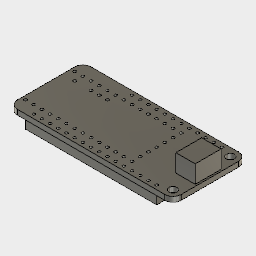
3200 Teensy Feather Adapter (Autodesk Fusion 360 design; units mm, degrees)
Autodesk Fusion 360 part; units mm, degrees
sketch "Adafruit Feather Teensy3 Adapter" plane through (0, 0, 0) normal (0, 0, 1) x (1, 0, 0)
  arc A0 (2.54, 22.86) -> (0, 20.32) centre (2.54, 20.32) ccw
  line L0 (2.54, 0) -> (48.26, 0)
  arc A1 (48.26, 0) -> (50.8, 2.54) centre (48.26, 2.54) ccw
  line L1 (48.26, 22.86) -> (2.54, 22.86)
  arc A2 (0, 2.54) -> (2.54, 0) centre (2.54, 2.54) ccw
  line L2 (0, 20.32) -> (0, 2.54)
  arc A3 (50.8, 20.32) -> (48.26, 22.86) centre (48.26, 20.32) ccw
  line L3 (50.8, 2.54) -> (50.8, 20.32)
  arc A4 (14.4145, 3.81) -> (13.5255, 3.81) centre (13.97, 3.81) ccw
  arc A5 (34.7345, 16.51) -> (33.8455, 16.51) centre (34.29, 16.51) ccw
  arc A6 (32.1945, 3.81) -> (31.3055, 3.81) centre (31.75, 3.81) ccw
  arc A7 (31.3055, 3.81) -> (32.1945, 3.81) centre (31.75, 3.81) ccw
  arc A8 (16.9545, 19.05) -> (16.0655, 19.05) centre (16.51, 19.05) ccw
  arc A9 (37.2491, 1.27) -> (36.4109, 1.27) centre (36.83, 1.27) ccw
  arc A10 (42.3291, 21.59) -> (41.4909, 21.59) centre (41.91, 21.59) ccw
  arc A11 (14.4145, 19.05) -> (13.5255, 19.05) centre (13.97, 19.05) ccw
  arc A12 (26.2255, 19.05) -> (27.1145, 19.05) centre (26.67, 19.05) ccw
  arc A13 (10.9855, 3.81) -> (11.8745, 3.81) centre (11.43, 3.81) ccw
  arc A14 (32.1945, 19.05) -> (31.3055, 19.05) centre (31.75, 19.05) ccw
  arc A15 (3.3655, 16.51) -> (4.2545, 16.51) centre (3.81, 16.51) ccw
  arc A16 (41.4909, 1.27) -> (42.3291, 1.27) centre (41.91, 1.27) ccw
  arc A17 (32.1691, 21.59) -> (31.3309, 21.59) centre (31.75, 21.59) ccw
  arc A18 (33.8709, 21.59) -> (34.7091, 21.59) centre (34.29, 21.59) ccw
  arc A19 (5.9055, 19.05) -> (6.7945, 19.05) centre (6.35, 19.05) ccw
  arc A20 (10.9855, 19.05) -> (11.8745, 19.05) centre (11.43, 19.05) ccw
  arc A21 (36.4109, 21.59) -> (37.2491, 21.59) centre (36.83, 21.59) ccw
  arc A22 (19.4691, 1.27) -> (18.6309, 1.27) centre (19.05, 1.27) ccw
  arc A23 (34.7345, 19.05) -> (33.8455, 19.05) centre (34.29, 19.05) ccw
  arc A24 (39.7891, 21.59) -> (38.9509, 21.59) centre (39.37, 21.59) ccw
  arc A25 (24.5491, 21.59) -> (23.7109, 21.59) centre (24.13, 21.59) ccw
  arc A26 (5.9309, 1.27) -> (6.7691, 1.27) centre (6.35, 1.27) ccw
  arc A27 (39.7891, 1.27) -> (38.9509, 1.27) centre (39.37, 1.27) ccw
  arc A28 (37.2491, 21.59) -> (36.4109, 21.59) centre (36.83, 21.59) ccw
  arc A29 (21.1455, 3.81) -> (22.0345, 3.81) centre (21.59, 3.81) ccw
  arc A30 (29.6545, 3.81) -> (28.7655, 3.81) centre (29.21, 3.81) ccw
  arc A31 (31.3055, 19.05) -> (32.1945, 19.05) centre (31.75, 19.05) ccw
  arc A32 (22.0091, 21.59) -> (21.1709, 21.59) centre (21.59, 21.59) ccw
  arc A33 (18.6309, 21.59) -> (19.4691, 21.59) centre (19.05, 21.59) ccw
  arc A34 (16.9291, 21.59) -> (16.0909, 21.59) centre (16.51, 21.59) ccw
  arc A35 (4.2545, 3.81) -> (3.3655, 3.81) centre (3.81, 3.81) ccw
  arc A36 (19.4691, 21.59) -> (18.6309, 21.59) centre (19.05, 21.59) ccw
  arc A37 (16.0909, 21.59) -> (16.9291, 21.59) centre (16.51, 21.59) ccw
  arc A38 (10.9855, 3.81) -> (11.8745, 3.81) centre (11.43, 3.81) ccw
  arc A39 (32.1691, 1.27) -> (31.3309, 1.27) centre (31.75, 1.27) ccw
  arc A40 (21.1709, 1.27) -> (22.0091, 1.27) centre (21.59, 1.27) ccw
  arc A41 (44.0309, 21.59) -> (44.8691, 21.59) centre (44.45, 21.59) ccw
  arc A42 (18.6055, 3.81) -> (19.4945, 3.81) centre (19.05, 3.81) ccw
  arc A43 (39.7891, 21.59) -> (38.9509, 21.59) centre (39.37, 21.59) ccw
  arc A44 (1.7145, 19.05) -> (0.8255, 19.05) centre (1.27, 19.05) ccw
  arc A45 (31.3055, 19.05) -> (32.1945, 19.05) centre (31.75, 19.05) ccw
  arc A46 (28.7909, 21.59) -> (29.6291, 21.59) centre (29.21, 21.59) ccw
  arc A47 (34.7091, 1.27) -> (33.8709, 1.27) centre (34.29, 1.27) ccw
  arc A48 (34.7091, 1.27) -> (33.8709, 1.27) centre (34.29, 1.27) ccw
  arc A49 (4.2545, 3.81) -> (3.3655, 3.81) centre (3.81, 3.81) ccw
  arc A50 (31.3309, 1.27) -> (32.1691, 1.27) centre (31.75, 1.27) ccw
  arc A51 (28.7909, 1.27) -> (29.6291, 1.27) centre (29.21, 1.27) ccw
  arc A52 (26.2509, 21.59) -> (27.0891, 21.59) centre (26.67, 21.59) ccw
  arc A53 (23.7109, 1.27) -> (24.5491, 1.27) centre (24.13, 1.27) ccw
  arc A54 (33.8455, 8.89) -> (34.7345, 8.89) centre (34.29, 8.89) ccw
  arc A55 (28.7909, 1.27) -> (29.6291, 1.27) centre (29.21, 1.27) ccw
  arc A56 (3.3655, 3.81) -> (4.2545, 3.81) centre (3.81, 3.81) ccw
  arc A57 (29.6291, 21.59) -> (28.7909, 21.59) centre (29.21, 21.59) ccw
  arc A58 (13.5509, 1.27) -> (14.3891, 1.27) centre (13.97, 1.27) ccw
  arc A59 (16.9291, 21.59) -> (16.0909, 21.59) centre (16.51, 21.59) ccw
  arc A60 (27.0891, 1.27) -> (26.2509, 1.27) centre (26.67, 1.27) ccw
  arc A61 (34.7345, 8.89) -> (33.8455, 8.89) centre (34.29, 8.89) ccw
  arc A62 (22.0091, 1.27) -> (21.1709, 1.27) centre (21.59, 1.27) ccw
  arc A63 (9.3345, 3.81) -> (8.4455, 3.81) centre (8.89, 3.81) ccw
  arc A64 (44.8691, 1.27) -> (44.0309, 1.27) centre (44.45, 1.27) ccw
  arc A65 (18.6309, 1.27) -> (19.4691, 1.27) centre (19.05, 1.27) ccw
  arc A66 (33.8709, 1.27) -> (34.7091, 1.27) centre (34.29, 1.27) ccw
  arc A67 (22.0091, 21.59) -> (21.1709, 21.59) centre (21.59, 21.59) ccw
  arc A68 (9.3091, 1.27) -> (8.4709, 1.27) centre (8.89, 1.27) ccw
  arc A69 (16.9291, 1.27) -> (16.0909, 1.27) centre (16.51, 1.27) ccw
  arc A70 (14.3891, 1.27) -> (13.5509, 1.27) centre (13.97, 1.27) ccw
  arc A71 (24.5491, 21.59) -> (23.7109, 21.59) centre (24.13, 21.59) ccw
  arc A72 (23.7109, 1.27) -> (24.5491, 1.27) centre (24.13, 1.27) ccw
  arc A73 (38.9509, 1.27) -> (39.7891, 1.27) centre (39.37, 1.27) ccw
  arc A74 (26.2509, 1.27) -> (27.0891, 1.27) centre (26.67, 1.27) ccw
  arc A75 (16.0909, 1.27) -> (16.9291, 1.27) centre (16.51, 1.27) ccw
  arc A76 (24.5491, 1.27) -> (23.7109, 1.27) centre (24.13, 1.27) ccw
  arc A77 (11.0109, 1.27) -> (11.8491, 1.27) centre (11.43, 1.27) ccw
  arc A78 (44.8691, 21.59) -> (44.0309, 21.59) centre (44.45, 21.59) ccw
  arc A79 (27.0891, 21.59) -> (26.2509, 21.59) centre (26.67, 21.59) ccw
  arc A80 (16.9291, 1.27) -> (16.0909, 1.27) centre (16.51, 1.27) ccw
  arc A81 (21.1709, 1.27) -> (22.0091, 1.27) centre (21.59, 1.27) ccw
  arc A82 (8.4709, 1.27) -> (9.3091, 1.27) centre (8.89, 1.27) ccw
  arc A83 (14.3891, 1.27) -> (13.5509, 1.27) centre (13.97, 1.27) ccw
  arc A84 (29.6291, 21.59) -> (28.7909, 21.59) centre (29.21, 21.59) ccw
  arc A85 (11.8745, 3.81) -> (10.9855, 3.81) centre (11.43, 3.81) ccw
  arc A86 (36.4109, 1.27) -> (37.2491, 1.27) centre (36.83, 1.27) ccw
  arc A87 (33.8455, 8.89) -> (34.7345, 8.89) centre (34.29, 8.89) ccw
  arc A88 (13.5509, 1.27) -> (14.3891, 1.27) centre (13.97, 1.27) ccw
  arc A89 (27.0891, 1.27) -> (26.2509, 1.27) centre (26.67, 1.27) ccw
  arc A90 (23.7109, 21.59) -> (24.5491, 21.59) centre (24.13, 21.59) ccw
  arc A91 (11.0109, 1.27) -> (11.8491, 1.27) centre (11.43, 1.27) ccw
  arc A92 (37.2491, 1.27) -> (36.4109, 1.27) centre (36.83, 1.27) ccw
  arc A93 (29.6291, 1.27) -> (28.7909, 1.27) centre (29.21, 1.27) ccw
  arc A94 (18.6309, 21.59) -> (19.4691, 21.59) centre (19.05, 21.59) ccw
  arc A95 (27.0891, 21.59) -> (26.2509, 21.59) centre (26.67, 21.59) ccw
  arc A96 (5.9309, 1.27) -> (6.7691, 1.27) centre (6.35, 1.27) ccw
  arc A97 (41.4909, 1.27) -> (42.3291, 1.27) centre (41.91, 1.27) ccw
  arc A98 (34.7345, 8.89) -> (33.8455, 8.89) centre (34.29, 8.89) ccw
  arc A99 (29.6291, 1.27) -> (28.7909, 1.27) centre (29.21, 1.27) ccw
  arc A100 (6.7691, 1.27) -> (5.9309, 1.27) centre (6.35, 1.27) ccw
  arc A101 (21.1709, 21.59) -> (22.0091, 21.59) centre (21.59, 21.59) ccw
  arc A102 (6.7691, 1.27) -> (5.9309, 1.27) centre (6.35, 1.27) ccw
  arc A103 (8.4709, 1.27) -> (9.3091, 1.27) centre (8.89, 1.27) ccw
  arc A104 (16.0909, 1.27) -> (16.9291, 1.27) centre (16.51, 1.27) ccw
  arc A105 (9.3091, 1.27) -> (8.4709, 1.27) centre (8.89, 1.27) ccw
  arc A106 (33.8455, 11.43) -> (34.7345, 11.43) centre (34.29, 11.43) ccw
  arc A107 (0.8255, 19.05) -> (1.7145, 19.05) centre (1.27, 19.05) ccw
  arc A108 (16.0655, 19.05) -> (16.9545, 19.05) centre (16.51, 19.05) ccw
  arc A109 (33.8455, 13.97) -> (34.7345, 13.97) centre (34.29, 13.97) ccw
  arc A110 (5.9055, 3.81) -> (6.7945, 3.81) centre (6.35, 3.81) ccw
  arc A111 (16.0655, 3.81) -> (16.9545, 3.81) centre (16.51, 3.81) ccw
  arc A112 (11.8491, 1.27) -> (11.0109, 1.27) centre (11.43, 1.27) ccw
  arc A113 (9.3345, 19.05) -> (8.4455, 19.05) centre (8.89, 19.05) ccw
  arc A114 (44.0309, 1.27) -> (44.8691, 1.27) centre (44.45, 1.27) ccw
  arc A115 (26.2509, 1.27) -> (27.0891, 1.27) centre (26.67, 1.27) ccw
  arc A116 (39.7891, 1.27) -> (38.9509, 1.27) centre (39.37, 1.27) ccw
  arc A117 (22.0345, 19.05) -> (21.1455, 19.05) centre (21.59, 19.05) ccw
  arc A118 (33.8455, 6.35) -> (34.7345, 6.35) centre (34.29, 6.35) ccw
  arc A119 (34.7091, 21.59) -> (33.8709, 21.59) centre (34.29, 21.59) ccw
  arc A120 (32.1691, 1.27) -> (31.3309, 1.27) centre (31.75, 1.27) ccw
  arc A121 (13.5255, 16.51) -> (14.4145, 16.51) centre (13.97, 16.51) ccw
  arc A122 (31.3309, 1.27) -> (32.1691, 1.27) centre (31.75, 1.27) ccw
  arc A123 (33.8455, 3.81) -> (34.7345, 3.81) centre (34.29, 3.81) ccw
  arc A124 (27.1145, 19.05) -> (26.2255, 19.05) centre (26.67, 19.05) ccw
  arc A125 (33.8455, 3.81) -> (34.7345, 3.81) centre (34.29, 3.81) ccw
  arc A126 (6.7945, 19.05) -> (5.9055, 19.05) centre (6.35, 19.05) ccw
  arc A127 (16.9545, 3.81) -> (16.0655, 3.81) centre (16.51, 3.81) ccw
  arc A128 (19.4691, 1.27) -> (18.6309, 1.27) centre (19.05, 1.27) ccw
  arc A129 (21.1455, 19.05) -> (22.0345, 19.05) centre (21.59, 19.05) ccw
  arc A130 (31.3055, 3.81) -> (32.1945, 3.81) centre (31.75, 3.81) ccw
  arc A131 (33.8455, 16.51) -> (34.7345, 16.51) centre (34.29, 16.51) ccw
  arc A132 (36.4109, 21.59) -> (37.2491, 21.59) centre (36.83, 21.59) ccw
  arc A133 (41.4909, 21.59) -> (42.3291, 21.59) centre (41.91, 21.59) ccw
  arc A134 (8.4455, 3.81) -> (9.3345, 3.81) centre (8.89, 3.81) ccw
  arc A135 (13.5255, 3.81) -> (14.4145, 3.81) centre (13.97, 3.81) ccw
  arc A136 (47.381, 2.54) -> (49.139, 2.54) centre (48.26, 2.54) ccw
  arc A137 (3.3655, 16.51) -> (4.2545, 16.51) centre (3.81, 16.51) ccw
  arc A138 (4.2545, 16.51) -> (3.3655, 16.51) centre (3.81, 16.51) ccw
  arc A139 (34.7345, 19.05) -> (33.8455, 19.05) centre (34.29, 19.05) ccw
  arc A140 (47.381, 20.32) -> (49.139, 20.32) centre (48.26, 20.32) ccw
  arc A141 (16.9545, 3.81) -> (16.0655, 3.81) centre (16.51, 3.81) ccw
  arc A142 (24.5745, 19.05) -> (23.6855, 19.05) centre (24.13, 19.05) ccw
  arc A143 (13.5255, 19.05) -> (14.4145, 19.05) centre (13.97, 19.05) ccw
  arc A144 (44.0309, 1.27) -> (44.8691, 1.27) centre (44.45, 1.27) ccw
  arc A145 (13.5255, 3.81) -> (14.4145, 3.81) centre (13.97, 3.81) ccw
  arc A146 (31.3309, 21.59) -> (32.1691, 21.59) centre (31.75, 21.59) ccw
  arc A147 (11.8745, 19.05) -> (10.9855, 19.05) centre (11.43, 19.05) ccw
  arc A148 (18.6055, 3.81) -> (19.4945, 3.81) centre (19.05, 3.81) ccw
  arc A149 (34.7345, 3.81) -> (33.8455, 3.81) centre (34.29, 3.81) ccw
  arc A150 (1.7145, 19.05) -> (0.8255, 19.05) centre (1.27, 19.05) ccw
  arc A151 (19.4945, 19.05) -> (18.6055, 19.05) centre (19.05, 19.05) ccw
  arc A152 (23.6855, 3.81) -> (24.5745, 3.81) centre (24.13, 3.81) ccw
  arc A153 (23.6855, 3.81) -> (24.5745, 3.81) centre (24.13, 3.81) ccw
  arc A154 (28.7655, 19.05) -> (29.6545, 19.05) centre (29.21, 19.05) ccw
  arc A155 (16.0909, 21.59) -> (16.9291, 21.59) centre (16.51, 21.59) ccw
  arc A156 (23.7109, 21.59) -> (24.5491, 21.59) centre (24.13, 21.59) ccw
  arc A157 (13.5255, 16.51) -> (14.4145, 16.51) centre (13.97, 16.51) ccw
  arc A158 (9.3345, 19.05) -> (8.4455, 19.05) centre (8.89, 19.05) ccw
  arc A159 (28.7655, 3.81) -> (29.6545, 3.81) centre (29.21, 3.81) ccw
  arc A160 (29.6545, 3.81) -> (28.7655, 3.81) centre (29.21, 3.81) ccw
  arc A161 (26.2255, 3.81) -> (27.1145, 3.81) centre (26.67, 3.81) ccw
  arc A162 (6.7945, 3.81) -> (5.9055, 3.81) centre (6.35, 3.81) ccw
  arc A163 (11.8491, 1.27) -> (11.0109, 1.27) centre (11.43, 1.27) ccw
  arc A164 (42.3291, 1.27) -> (41.4909, 1.27) centre (41.91, 1.27) ccw
  arc A165 (8.4455, 19.05) -> (9.3345, 19.05) centre (8.89, 19.05) ccw
  arc A166 (0.8255, 3.81) -> (1.7145, 3.81) centre (1.27, 3.81) ccw
  arc A167 (33.8709, 1.27) -> (34.7091, 1.27) centre (34.29, 1.27) ccw
  arc A168 (44.8691, 1.27) -> (44.0309, 1.27) centre (44.45, 1.27) ccw
  arc A169 (21.1455, 19.05) -> (22.0345, 19.05) centre (21.59, 19.05) ccw
  arc A170 (28.7909, 21.59) -> (29.6291, 21.59) centre (29.21, 21.59) ccw
  arc A171 (6.7945, 3.81) -> (5.9055, 3.81) centre (6.35, 3.81) ccw
  arc A172 (4.2545, 19.05) -> (3.3655, 19.05) centre (3.81, 19.05) ccw
  arc A173 (49.139, 2.54) -> (47.381, 2.54) centre (48.26, 2.54) ccw
  arc A174 (16.0655, 19.05) -> (16.9545, 19.05) centre (16.51, 19.05) ccw
  arc A175 (14.4145, 3.81) -> (13.5255, 3.81) centre (13.97, 3.81) ccw
  arc A176 (18.6055, 19.05) -> (19.4945, 19.05) centre (19.05, 19.05) ccw
  arc A177 (34.7345, 13.97) -> (33.8455, 13.97) centre (34.29, 13.97) ccw
  arc A178 (34.7345, 11.43) -> (33.8455, 11.43) centre (34.29, 11.43) ccw
  arc A179 (14.4145, 19.05) -> (13.5255, 19.05) centre (13.97, 19.05) ccw
  arc A180 (21.1455, 3.81) -> (22.0345, 3.81) centre (21.59, 3.81) ccw
  arc A181 (0.8255, 19.05) -> (1.7145, 19.05) centre (1.27, 19.05) ccw
  arc A182 (32.1691, 21.59) -> (31.3309, 21.59) centre (31.75, 21.59) ccw
  arc A183 (33.8455, 19.05) -> (34.7345, 19.05) centre (34.29, 19.05) ccw
  arc A184 (34.7345, 11.43) -> (33.8455, 11.43) centre (34.29, 11.43) ccw
  arc A185 (16.9545, 19.05) -> (16.0655, 19.05) centre (16.51, 19.05) ccw
  arc A186 (16.0655, 3.81) -> (16.9545, 3.81) centre (16.51, 3.81) ccw
  arc A187 (14.4145, 16.51) -> (13.5255, 16.51) centre (13.97, 16.51) ccw
  arc A188 (24.5745, 3.81) -> (23.6855, 3.81) centre (24.13, 3.81) ccw
  arc A189 (34.7345, 16.51) -> (33.8455, 16.51) centre (34.29, 16.51) ccw
  arc A190 (22.0091, 1.27) -> (21.1709, 1.27) centre (21.59, 1.27) ccw
  arc A191 (33.8709, 21.59) -> (34.7091, 21.59) centre (34.29, 21.59) ccw
  arc A192 (3.3655, 3.81) -> (4.2545, 3.81) centre (3.81, 3.81) ccw
  arc A193 (26.2509, 21.59) -> (27.0891, 21.59) centre (26.67, 21.59) ccw
  arc A194 (19.4691, 21.59) -> (18.6309, 21.59) centre (19.05, 21.59) ccw
  arc A195 (24.5745, 3.81) -> (23.6855, 3.81) centre (24.13, 3.81) ccw
  arc A196 (33.8455, 19.05) -> (34.7345, 19.05) centre (34.29, 19.05) ccw
  arc A197 (34.7345, 13.97) -> (33.8455, 13.97) centre (34.29, 13.97) ccw
  arc A198 (49.139, 2.54) -> (47.381, 2.54) centre (48.26, 2.54) ccw
  arc A199 (38.9509, 1.27) -> (39.7891, 1.27) centre (39.37, 1.27) ccw
  arc A200 (9.3345, 16.51) -> (8.4455, 16.51) centre (8.89, 16.51) ccw
  arc A201 (11.8745, 19.05) -> (10.9855, 19.05) centre (11.43, 19.05) ccw
  arc A202 (32.1945, 3.81) -> (31.3055, 3.81) centre (31.75, 3.81) ccw
  arc A203 (29.6545, 19.05) -> (28.7655, 19.05) centre (29.21, 19.05) ccw
  arc A204 (10.9855, 16.51) -> (11.8745, 16.51) centre (11.43, 16.51) ccw
  arc A205 (33.8455, 16.51) -> (34.7345, 16.51) centre (34.29, 16.51) ccw
  arc A206 (26.2255, 19.05) -> (27.1145, 19.05) centre (26.67, 19.05) ccw
  arc A207 (9.3345, 3.81) -> (8.4455, 3.81) centre (8.89, 3.81) ccw
  arc A208 (5.9055, 3.81) -> (6.7945, 3.81) centre (6.35, 3.81) ccw
  arc A209 (34.7345, 6.35) -> (33.8455, 6.35) centre (34.29, 6.35) ccw
  arc A210 (21.1709, 21.59) -> (22.0091, 21.59) centre (21.59, 21.59) ccw
  arc A211 (23.6855, 19.05) -> (24.5745, 19.05) centre (24.13, 19.05) ccw
  arc A212 (34.7091, 21.59) -> (33.8709, 21.59) centre (34.29, 21.59) ccw
  arc A213 (5.9055, 19.05) -> (6.7945, 19.05) centre (6.35, 19.05) ccw
  arc A214 (1.7145, 3.81) -> (0.8255, 3.81) centre (1.27, 3.81) ccw
  arc A215 (49.139, 20.32) -> (47.381, 20.32) centre (48.26, 20.32) ccw
  arc A216 (10.9855, 19.05) -> (11.8745, 19.05) centre (11.43, 19.05) ccw
  arc A217 (28.7655, 3.81) -> (29.6545, 3.81) centre (29.21, 3.81) ccw
  arc A218 (11.8745, 16.51) -> (10.9855, 16.51) centre (11.43, 16.51) ccw
  arc A219 (11.8745, 16.51) -> (10.9855, 16.51) centre (11.43, 16.51) ccw
  arc A220 (41.4909, 21.59) -> (42.3291, 21.59) centre (41.91, 21.59) ccw
  arc A221 (29.6545, 19.05) -> (28.7655, 19.05) centre (29.21, 19.05) ccw
  arc A222 (34.7345, 3.81) -> (33.8455, 3.81) centre (34.29, 3.81) ccw
  arc A223 (8.4455, 19.05) -> (9.3345, 19.05) centre (8.89, 19.05) ccw
  arc A224 (27.1145, 3.81) -> (26.2255, 3.81) centre (26.67, 3.81) ccw
  arc A225 (44.8691, 21.59) -> (44.0309, 21.59) centre (44.45, 21.59) ccw
  arc A226 (34.7345, 6.35) -> (33.8455, 6.35) centre (34.29, 6.35) ccw
  arc A227 (33.8455, 11.43) -> (34.7345, 11.43) centre (34.29, 11.43) ccw
  arc A228 (28.7655, 19.05) -> (29.6545, 19.05) centre (29.21, 19.05) ccw
  arc A229 (22.0345, 3.81) -> (21.1455, 3.81) centre (21.59, 3.81) ccw
  arc A230 (37.2491, 21.59) -> (36.4109, 21.59) centre (36.83, 21.59) ccw
  arc A231 (19.4945, 19.05) -> (18.6055, 19.05) centre (19.05, 19.05) ccw
  arc A232 (19.4945, 3.81) -> (18.6055, 3.81) centre (19.05, 3.81) ccw
  arc A233 (44.0309, 21.59) -> (44.8691, 21.59) centre (44.45, 21.59) ccw
  arc A234 (3.3655, 19.05) -> (4.2545, 19.05) centre (3.81, 19.05) ccw
  arc A235 (19.4945, 3.81) -> (18.6055, 3.81) centre (19.05, 3.81) ccw
  arc A236 (18.6309, 1.27) -> (19.4691, 1.27) centre (19.05, 1.27) ccw
  arc A237 (8.4455, 16.51) -> (9.3345, 16.51) centre (8.89, 16.51) ccw
  arc A238 (33.8455, 6.35) -> (34.7345, 6.35) centre (34.29, 6.35) ccw
  arc A239 (33.8455, 13.97) -> (34.7345, 13.97) centre (34.29, 13.97) ccw
  arc A240 (10.9855, 16.51) -> (11.8745, 16.51) centre (11.43, 16.51) ccw
  arc A241 (47.381, 2.54) -> (49.139, 2.54) centre (48.26, 2.54) ccw
  arc A242 (36.4109, 1.27) -> (37.2491, 1.27) centre (36.83, 1.27) ccw
  arc A243 (47.381, 20.32) -> (49.139, 20.32) centre (48.26, 20.32) ccw
  arc A244 (6.7945, 19.05) -> (5.9055, 19.05) centre (6.35, 19.05) ccw
  arc A245 (26.2255, 3.81) -> (27.1145, 3.81) centre (26.67, 3.81) ccw
  arc A246 (13.5255, 19.05) -> (14.4145, 19.05) centre (13.97, 19.05) ccw
  arc A247 (42.3291, 1.27) -> (41.4909, 1.27) centre (41.91, 1.27) ccw
  arc A248 (22.0345, 3.81) -> (21.1455, 3.81) centre (21.59, 3.81) ccw
  arc A249 (27.1145, 3.81) -> (26.2255, 3.81) centre (26.67, 3.81) ccw
  arc A250 (24.5745, 19.05) -> (23.6855, 19.05) centre (24.13, 19.05) ccw
  arc A251 (14.4145, 16.51) -> (13.5255, 16.51) centre (13.97, 16.51) ccw
  arc A252 (22.0345, 19.05) -> (21.1455, 19.05) centre (21.59, 19.05) ccw
  arc A253 (49.139, 20.32) -> (47.381, 20.32) centre (48.26, 20.32) ccw
  arc A254 (38.9509, 21.59) -> (39.7891, 21.59) centre (39.37, 21.59) ccw
  arc A255 (42.3291, 21.59) -> (41.4909, 21.59) centre (41.91, 21.59) ccw
  arc A256 (3.3655, 19.05) -> (4.2545, 19.05) centre (3.81, 19.05) ccw
  arc A257 (9.3345, 16.51) -> (8.4455, 16.51) centre (8.89, 16.51) ccw
  arc A258 (18.6055, 19.05) -> (19.4945, 19.05) centre (19.05, 19.05) ccw
  arc A259 (38.9509, 21.59) -> (39.7891, 21.59) centre (39.37, 21.59) ccw
  arc A260 (0.8255, 3.81) -> (1.7145, 3.81) centre (1.27, 3.81) ccw
  arc A261 (31.3309, 21.59) -> (32.1691, 21.59) centre (31.75, 21.59) ccw
  arc A262 (32.1945, 19.05) -> (31.3055, 19.05) centre (31.75, 19.05) ccw
  arc A263 (1.7145, 3.81) -> (0.8255, 3.81) centre (1.27, 3.81) ccw
  arc A264 (24.5491, 1.27) -> (23.7109, 1.27) centre (24.13, 1.27) ccw
  arc A265 (23.6855, 19.05) -> (24.5745, 19.05) centre (24.13, 19.05) ccw
  arc A266 (8.4455, 3.81) -> (9.3345, 3.81) centre (8.89, 3.81) ccw
  arc A267 (11.8745, 3.81) -> (10.9855, 3.81) centre (11.43, 3.81) ccw
  arc A268 (27.1145, 19.05) -> (26.2255, 19.05) centre (26.67, 19.05) ccw
  arc A269 (4.2545, 16.51) -> (3.3655, 16.51) centre (3.81, 16.51) ccw
  arc A270 (8.4455, 16.51) -> (9.3345, 16.51) centre (8.89, 16.51) ccw
  arc A271 (4.2545, 19.05) -> (3.3655, 19.05) centre (3.81, 19.05) ccw
  circle A272 centre (48.26, 20.32) radius 1.27
  circle A273 centre (48.26, 2.54) radius 1.25
  dimension "d3" = 2.54
  dimension "d4" = 2.5
  measures "d3" diameter of A272
  measures "d4" diameter of A273
extrude "Extrude1" add sketch "Adafruit Feather Teensy3 Adapter" along normal blind 1.6 contours A0 L0 A1 L1 A2 L2 A3 L3 makes body 1
sketch "Sketch2" plane through (0, 0, 1.6) normal (0, 0, 1) x (-1, 0, 0)
  circle A0 centre (-21.59, -1.27) radius 0.4191
  circle A1 centre (-34.29, -21.59) radius 0.4191
  circle A2 centre (-19.05, -19.05) radius 0.4445
  circle A3 centre (-41.91, -21.59) radius 0.4191
  circle A4 centre (-13.97, -16.51) radius 0.4445
  circle A5 centre (-8.89, -19.05) radius 0.4445
  circle A6 centre (-6.35, -19.05) radius 0.4445
  circle A7 centre (-13.97, -3.81) radius 0.4445
  circle A8 centre (-21.59, -3.81) radius 0.4445
  circle A9 centre (-44.45, -21.59) radius 0.4191
  circle A10 centre (-1.27, -19.05) radius 0.4445
  circle A11 centre (-21.59, -21.59) radius 0.4191
  circle A12 centre (-48.26, -2.54) radius 1.25
  circle A13 centre (-26.67, -21.59) radius 0.4191
  circle A14 centre (-34.29, -16.51) radius 0.4445
  circle A15 centre (-34.29, -19.05) radius 0.4445
  circle A16 centre (-11.43, -3.81) radius 0.4445
  circle A17 centre (-11.43, -19.05) radius 0.4445
  circle A18 centre (-24.13, -1.27) radius 0.4191
  circle A19 centre (-16.51, -3.81) radius 0.4445
  circle A20 centre (-11.43, -16.51) radius 0.4445
  circle A21 centre (-21.59, -19.05) radius 0.4445
  circle A22 centre (-13.97, -19.05) radius 0.4445
  circle A23 centre (-36.83, -21.59) radius 0.4191
  circle A24 centre (-6.35, -3.81) radius 0.4445
  circle A25 centre (-36.83, -1.27) radius 0.4191
  circle A26 centre (-39.37, -21.59) radius 0.4191
  circle A27 centre (-24.13, -21.59) radius 0.4191
  circle A28 centre (-41.91, -1.27) radius 0.4191
  circle A29 centre (-11.43, -1.27) radius 0.4191
  circle A30 centre (-6.35, -1.27) radius 0.4191
  circle A31 centre (-13.97, -1.27) radius 0.4191
  circle A32 centre (-29.21, -1.27) radius 0.4191
  circle A33 centre (-34.29, -8.89) radius 0.4445
  circle A34 centre (-16.51, -1.27) radius 0.4191
  circle A35 centre (-8.89, -1.27) radius 0.4191
  circle A36 centre (-26.67, -1.27) radius 0.4191
  circle A37 centre (-31.75, -1.27) radius 0.4191
  circle A38 centre (-16.51, -21.59) radius 0.4191
  circle A39 centre (-34.29, -3.81) radius 0.4445
  circle A40 centre (-48.26, -20.32) radius 1.27
  circle A41 centre (-26.67, -3.81) radius 0.4445
  circle A42 centre (-29.21, -19.05) radius 0.4445
  circle A43 centre (-19.05, -21.59) radius 0.4191
  circle A44 centre (-24.13, -3.81) radius 0.4445
  circle A45 centre (-24.13, -19.05) radius 0.4445
  circle A46 centre (-44.45, -1.27) radius 0.4191
  circle A47 centre (-29.21, -21.59) radius 0.4191
  circle A48 centre (-26.67, -19.05) radius 0.4445
  circle A49 centre (-16.51, -19.05) radius 0.4445
  circle A50 centre (-8.89, -3.81) radius 0.4445
  circle A51 centre (-19.05, -1.27) radius 0.4191
  circle A52 centre (-1.27, -3.81) radius 0.4445
  circle A53 centre (-34.29, -11.43) radius 0.4445
  circle A54 centre (-39.37, -1.27) radius 0.4191
  circle A55 centre (-19.05, -3.81) radius 0.4445
  circle A56 centre (-3.81, -19.05) radius 0.4445
  circle A57 centre (-31.75, -19.05) radius 0.4445
  circle A58 centre (-34.29, -6.35) radius 0.4445
  circle A59 centre (-34.29, -13.97) radius 0.4445
  circle A60 centre (-31.75, -3.81) radius 0.4445
  circle A61 centre (-29.21, -3.81) radius 0.4445
  circle A62 centre (-31.75, -21.59) radius 0.4191
  circle A63 centre (-3.81, -16.51) radius 0.4445
  circle A64 centre (-34.29, -1.27) radius 0.4191
  circle A65 centre (-8.89, -16.51) radius 0.4445
  circle A66 centre (-3.81, -3.81) radius 0.4445
  line L0 (-50.8, -2.54) -> (-50.8, -20.32)
  arc A67 (-50.8, -20.32) -> (-48.26, -22.86) centre (-48.26, -20.32) ccw
  line L1 (-48.26, -22.86) -> (-2.54, -22.86)
  arc A68 (-2.54, -22.86) -> (0, -20.32) centre (-2.54, -20.32) ccw
  line L2 (0, -20.32) -> (0, -2.54)
  arc A69 (0, -2.54) -> (-2.54, 0) centre (-2.54, -2.54) ccw
  line L3 (-2.54, 0) -> (-48.26, 0)
  arc A70 (-48.26, 0) -> (-50.8, -2.54) centre (-48.26, -2.54) ccw
  line L4 (-50.8, -11.43) -> (0, -11.43) construction
  line L5 (-50.244, -7.43) -> (-44.244, -7.43)
  line L6 (-44.244, -7.43) -> (-44.244, -15.43)
  line L7 (-44.244, -15.43) -> (-50.244, -15.43)
  line L8 (-50.244, -15.43) -> (-50.244, -7.43)
  line L9 (-50.244, -7.43) -> (-44.244, -15.43) construction
  line L10 (-44.244, -7.43) -> (-50.244, -15.43) construction
  point P0 (-47.244, -11.43)
  dimension "d5" = 6
  dimension "d6" = 8
  dimension "d7" = 47.244
  measures "d5" distance of L6.end L7.end
  measures "d6" distance of L5.end L6.end
  measures "d7" distance of L2 P0
extrude "Extrude2" add sketch "Sketch2" along normal blind 5.5 separate body contours L5 L6 L7 L8 makes body 2
sketch "Sketch3" plane through (0, 0, 0) normal (0, 0, -1) x (1, 0, 0)
  circle A0 centre (21.59, -1.27) radius 0.4191
  circle A1 centre (34.29, -21.59) radius 0.4191
  circle A2 centre (19.05, -19.05) radius 0.4445
  circle A3 centre (41.91, -21.59) radius 0.4191
  circle A4 centre (13.97, -16.51) radius 0.4445
  circle A5 centre (8.89, -19.05) radius 0.4445
  circle A6 centre (6.35, -19.05) radius 0.4445
  circle A7 centre (13.97, -3.81) radius 0.4445
  circle A8 centre (21.59, -3.81) radius 0.4445
  circle A9 centre (44.45, -21.59) radius 0.4191
  circle A10 centre (1.27, -19.05) radius 0.4445
  circle A11 centre (21.59, -21.59) radius 0.4191
  circle A12 centre (48.26, -2.54) radius 1.25
  circle A13 centre (26.67, -21.59) radius 0.4191
  circle A14 centre (34.29, -16.51) radius 0.4445
  circle A15 centre (34.29, -19.05) radius 0.4445
  circle A16 centre (11.43, -3.81) radius 0.4445
  circle A17 centre (11.43, -19.05) radius 0.4445
  circle A18 centre (24.13, -1.27) radius 0.4191
  circle A19 centre (16.51, -3.81) radius 0.4445
  circle A20 centre (11.43, -16.51) radius 0.4445
  circle A21 centre (21.59, -19.05) radius 0.4445
  circle A22 centre (13.97, -19.05) radius 0.4445
  circle A23 centre (36.83, -21.59) radius 0.4191
  circle A24 centre (6.35, -3.81) radius 0.4445
  circle A25 centre (36.83, -1.27) radius 0.4191
  circle A26 centre (39.37, -21.59) radius 0.4191
  circle A27 centre (24.13, -21.59) radius 0.4191
  circle A28 centre (41.91, -1.27) radius 0.4191
  circle A29 centre (11.43, -1.27) radius 0.4191
  circle A30 centre (6.35, -1.27) radius 0.4191
  circle A31 centre (13.97, -1.27) radius 0.4191
  circle A32 centre (29.21, -1.27) radius 0.4191
  circle A33 centre (34.29, -8.89) radius 0.4445
  circle A34 centre (16.51, -1.27) radius 0.4191
  circle A35 centre (8.89, -1.27) radius 0.4191
  circle A36 centre (26.67, -1.27) radius 0.4191
  circle A37 centre (31.75, -1.27) radius 0.4191
  circle A38 centre (16.51, -21.59) radius 0.4191
  circle A39 centre (34.29, -3.81) radius 0.4445
  circle A40 centre (48.26, -20.32) radius 1.27
  circle A41 centre (26.67, -3.81) radius 0.4445
  circle A42 centre (29.21, -19.05) radius 0.4445
  circle A43 centre (19.05, -21.59) radius 0.4191
  circle A44 centre (24.13, -3.81) radius 0.4445
  circle A45 centre (24.13, -19.05) radius 0.4445
  circle A46 centre (44.45, -1.27) radius 0.4191
  circle A47 centre (29.21, -21.59) radius 0.4191
  circle A48 centre (26.67, -19.05) radius 0.4445
  circle A49 centre (16.51, -19.05) radius 0.4445
  circle A50 centre (8.89, -3.81) radius 0.4445
  circle A51 centre (19.05, -1.27) radius 0.4191
  circle A52 centre (1.27, -3.81) radius 0.4445
  circle A53 centre (34.29, -11.43) radius 0.4445
  circle A54 centre (39.37, -1.27) radius 0.4191
  circle A55 centre (19.05, -3.81) radius 0.4445
  circle A56 centre (3.81, -19.05) radius 0.4445
  circle A57 centre (31.75, -19.05) radius 0.4445
  circle A58 centre (34.29, -6.35) radius 0.4445
  circle A59 centre (34.29, -13.97) radius 0.4445
  circle A60 centre (31.75, -3.81) radius 0.4445
  circle A61 centre (29.21, -3.81) radius 0.4445
  circle A62 centre (31.75, -21.59) radius 0.4191
  circle A63 centre (3.81, -16.51) radius 0.4445
  circle A64 centre (34.29, -1.27) radius 0.4191
  circle A65 centre (8.89, -16.51) radius 0.4445
  circle A66 centre (3.81, -3.81) radius 0.4445
  line L0 (50.8, -20.32) -> (50.8, -2.54)
  arc A67 (50.8, -2.54) -> (48.26, 0) centre (48.26, -2.54) ccw
  line L1 (48.26, 0) -> (2.54, 0)
  arc A68 (2.54, 0) -> (0, -2.54) centre (2.54, -2.54) ccw
  line L2 (0, -2.54) -> (0, -20.32)
  arc A69 (0, -20.32) -> (2.54, -22.86) centre (2.54, -20.32) ccw
  line L3 (2.54, -22.86) -> (48.26, -22.86)
  arc A70 (48.26, -22.86) -> (50.8, -20.32) centre (48.26, -20.32) ccw
  line L4 (5.08, 0) -> (45.72, 0)
  line L5 (45.72, 0) -> (45.72, -2.54)
  line L6 (45.72, -2.54) -> (5.08, -2.54)
  line L7 (5.08, -2.54) -> (5.08, 0)
  line L8 (45.72, -20.32) -> (15.24, -20.32)
  line L9 (15.24, -20.32) -> (15.24, -22.86)
  line L10 (15.24, -22.86) -> (45.72, -22.86)
  line L11 (45.72, -22.86) -> (45.72, -20.32)
  dimension "d10" = 1.27
  dimension "d11" = 1.27
  dimension "d12" = 1.27
  dimension "d13" = 1.27
  dimension "d14" = 1.27
  dimension "d15" = 1.27
  measures "d10" distance of A46.centre L6
  measures "d11" distance of A46.centre L5
  measures "d12" distance of A30.centre L7
  measures "d13" distance of A38.centre L9
  measures "d14" distance of A38.centre L8
  measures "d15" distance of A9.centre L11
extrude "Extrude3" add sketch "Sketch3" along normal blind 2.5 separate body contours L3 L8 L9 L10 L11 | L1 L4 L5 L6 L7 makes body 3 at (35.56, 20.32, -0.8333) makes body 4 at (32.1733, 2.54, -1.6667)
